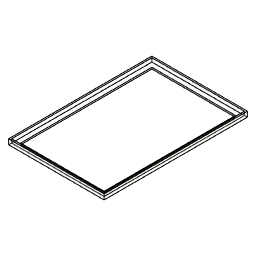
SafetyMachineCase (Autodesk Fusion 360 archive; units mm, degrees)
design "cover"
Autodesk Fusion 360 part; units mm, degrees
(part 1 of 2)
sketch "スケッチ1" plane through (0, 0, 0) normal (0, 0, 1) x (1, 0, 0)
  line L0 (31, 47) -> (-31, 47)
  line L1 (-31, 47) -> (-31, -47)
  line L2 (-31, -47) -> (31, -47)
  line L3 (31, -47) -> (31, 47)
  line L4 (31, 47) -> (-31, -47) construction
  line L5 (-31, 47) -> (31, -47) construction
  line L6 (-32, 48) -> (-32, -48)
  line L7 (-32, -48) -> (32, -48)
  line L8 (32, -48) -> (32, 48)
  line L9 (32, 48) -> (-32, 48)
  line L10 (-28, 44) -> (-28, -44)
  line L11 (-28, -44) -> (28, -44)
  line L12 (28, -44) -> (28, 44)
  line L13 (28, 44) -> (-28, 44)
  dimension "d1" = 62
  dimension "d2" = 94
  dimension "d3" = 1
  dimension "d4" = -3
  constraint horizontal L0
  constraint perpendicular L0 L1
  constraint parallel L0 L2
  constraint parallel L1 L3
  constraint coincident L4 origin
  constraint coincident L5 origin
  measures "d1" distance of L0.start L0.end
  measures "d2" distance of L0.start L2.end
extrude "押し出し1" add sketch "スケッチ1" along normal blind 2.5 contours L6 L7 L8 L9
extrude "押し出し2" add sketch "スケッチ1" against normal blind 1 contours L0 L1 L2 L3 | L6 L7 L8 L9

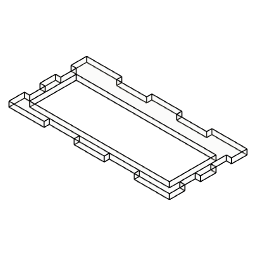
design "migisokumen"
Autodesk Fusion 360 part; units mm, degrees
sketch "スケッチ1" plane through (0, 0, 0) normal (0, 0, 1) x (1, 0, 0)
  line L0 (31, 15) -> (-31, 15)
  line L1 (-31, 15) -> (-31, -15)
  line L2 (-31, -15) -> (31, -15)
  line L3 (31, -15) -> (31, 15)
  line L4 (31, 15) -> (-31, -15) construction
  line L5 (-31, 15) -> (31, -15) construction
  dimension "d1" = 62
  dimension "d2" = 30
  constraint horizontal L0
  constraint perpendicular L0 L1
  constraint parallel L0 L2
  constraint parallel L1 L3
  constraint coincident L4 origin
  constraint coincident L5 origin
  measures "d1" distance of L0.start L0.end
  measures "d2" distance of L0.end L1.end
extrude "押し出し1" add sketch "スケッチ1" along normal blind 2
sketch "スケッチ2" plane through (0, 0, 0) normal (0, 0, 1) x (1, 0, 0)
  line L0 (31, 9) -> (29, 9)
  line L1 (29, 9) -> (29, 3)
  line L2 (29, 3) -> (31, 3)
  line L3 (31, 3) -> (31, 9)
  line L4 (31, -15) -> (31, 15)
  line L5 (0, 0) -> (48, 0)
  line L6 (31, -3) -> (31, -9)
  line L7 (29, -3) -> (31, -3)
  line L8 (29, -9) -> (29, -3)
  line L9 (31, -9) -> (29, -9)
  line L10 (0, 0) -> (0, -25)
  line L11 (-31, 9) -> (-29, 9)
  line L12 (-31, 3) -> (-31, 9)
  line L13 (-29, -3) -> (-31, -3)
  line L14 (-31, -3) -> (-31, -9)
  line L15 (-31, -9) -> (-29, -9)
  line L16 (-29, -9) -> (-29, -3)
  line L17 (-29, 3) -> (-31, 3)
  line L18 (-29, 9) -> (-29, 3)
  dimension "d9" = 6
  dimension "d10" = 3
  dimension "d23" = 2
  constraint horizontal L0
  constraint vertical L1
  constraint horizontal L2
  constraint vertical L3
  constraint collinear L3 L4
  constraint coincident L5.start L10.start
  constraint perpendicular L4 L5
  constraint symmetric L0.start L5 L6.end
  constraint symmetric L0.end L5 L8.start
  constraint symmetric L1.end L5 L7.start
  constraint symmetric L2.end L5 L6.start
  constraint perpendicular L5 L10
  constraint symmetric L0.start L10 L11.start
  constraint symmetric L0.end L10 L11.end
  constraint symmetric L1.end L10 L17.start
  constraint symmetric L2.end L10 L12.start
  constraint symmetric L8.start L10 L15.end
  constraint symmetric L6.end L10 L14.end
  constraint symmetric L6.start L10 L13.end
  constraint symmetric L7.start L10 L13.start
  measures "d9" distance of L0.end L1.end
  measures "d10" distance of L5.start L2
  measures "d23" distance of L1 L3
extrude "押し出し2" cut sketch "スケッチ2" along normal up to surface (2 mm away)
sketch "スケッチ3" plane through (0, 0, 2) normal (0, 0, 1) x (-1, 0, 0)
  line L0 (-31, 3) -> (-31, -3)
  line L1 (-31, -15) -> (31, -15)
  line L2 (31, -15) -> (31, -9)
  line L3 (17.4, -15) -> (5.8, -15)
  line L4 (5.8, -15) -> (5.8, -13)
  line L5 (5.8, -13) -> (17.4, -13)
  line L6 (17.4, -13) -> (17.4, -15)
  line L7 (0, 0) -> (0, -10)
  line L8 (0, 0) -> (9, 0)
  line L9 (-17.4, -15) -> (-5.8, -15)
  line L10 (-5.8, -15) -> (-5.8, -13)
  line L11 (-17.4, -13) -> (-17.4, -15)
  line L12 (-5.8, -13) -> (-17.4, -13)
  line L13 (-5.8, 15) -> (-5.8, 13)
  line L14 (-17.4, 13) -> (-17.4, 15)
  line L15 (17.4, 15) -> (5.8, 15)
  line L16 (5.8, 13) -> (17.4, 13)
  line L17 (-17.4, 15) -> (-5.8, 15)
  line L18 (-5.8, 13) -> (-17.4, 13)
  line L19 (5.8, 15) -> (5.8, 13)
  line L20 (17.4, 13) -> (17.4, 15)
  line L21 (-31, 9) -> (-29, 9)
  line L22 (-29, 9) -> (-29, 3)
  line L23 (-29, 3) -> (-31, 3)
  line L24 (-31, -3) -> (-29, -3)
  line L25 (-29, -3) -> (-29, -9)
  line L26 (-29, -9) -> (-31, -9)
  line L27 (-31, -9) -> (-31, -15)
  line L28 (31, -9) -> (29, -9)
  line L29 (29, -9) -> (29, -3)
  line L30 (29, -3) -> (31, -3)
  line L31 (31, -3) -> (31, 3)
  line L32 (31, 3) -> (29, 3)
  line L33 (29, 3) -> (29, 9)
  line L34 (29, 9) -> (31, 9)
  line L35 (31, 9) -> (31, 15)
  line L36 (-31, 15) -> (-31, 9)
  dimension "d16" = 11.6
  dimension "d21" = 2
  dimension "d22" = 5.8
  constraint horizontal L3
  constraint vertical L4
  constraint horizontal L5
  constraint vertical L6
  constraint coincident L1 L3.start
  constraint coincident L7.start L8.start
  constraint parallel L4 L7
  constraint perpendicular L7 L8
  constraint symmetric L3.start L7 L9.start
  constraint symmetric L3.end L7 L9.end
  constraint symmetric L4.end L7 L10.end
  constraint symmetric L5.end L7 L11.start
  constraint symmetric L3.start L8 L15.start
  constraint symmetric L3.end L8 L15.end
  constraint symmetric L4.end L8 L16.start
  constraint symmetric L5.end L8 L16.end
  constraint symmetric L8 L9.start L14.end
  constraint symmetric L8 L9.end L13.start
  constraint symmetric L8 L11.start L14.start
  constraint symmetric L8 L10.end L13.end
  measures "d16" distance of L4.end L5.end
  measures "d21" distance of L1 L5
  measures "d22" distance of L7.start L4
extrude "押し出し3" cut sketch "スケッチ3" against normal up to surface (2 mm away)
sketch "スケッチ4" plane through (0, 0, 2) normal (0, 0, 1) x (-1, 0, 0)
  line L0 (-17.4, -15) -> (-17.4, -13)
  line L1 (-17.4, -13) -> (-5.8, -13)
  line L2 (-5.8, -13) -> (-5.8, -15)
  line L3 (-5.8, -15) -> (5.8, -15)
  line L4 (5.8, -15) -> (5.8, -13)
  line L5 (5.8, -13) -> (17.4, -13)
  line L6 (17.4, -13) -> (17.4, -15)
  line L7 (17.4, -15) -> (31, -15)
  line L8 (31, -15) -> (31, -9)
  line L9 (31, -9) -> (29, -9)
  line L10 (29, -9) -> (29, -3)
  line L11 (29, -3) -> (31, -3)
  line L12 (31, -3) -> (31, 3)
  line L13 (31, 3) -> (29, 3)
  line L14 (29, 3) -> (29, 9)
  line L15 (29, 9) -> (31, 9)
  line L16 (31, 9) -> (31, 15)
  line L17 (31, 15) -> (17.4, 15)
  line L18 (17.4, 15) -> (17.4, 13)
  line L19 (17.4, 13) -> (5.8, 13)
  line L20 (5.8, 13) -> (5.8, 15)
  line L21 (5.8, 15) -> (-5.8, 15)
  line L22 (-5.8, 15) -> (-5.8, 13)
  line L23 (-5.8, 13) -> (-17.4, 13)
  line L24 (-17.4, 13) -> (-17.4, 15)
  line L25 (-17.4, 15) -> (-31, 15)
  line L26 (-31, 15) -> (-31, 9)
  line L27 (-31, 9) -> (-29, 9)
  line L28 (-29, 9) -> (-29, 3)
  line L29 (-29, 3) -> (-31, 3)
  line L30 (-31, 3) -> (-31, -3)
  line L31 (-31, -3) -> (-29, -3)
  line L32 (-29, -3) -> (-29, -9)
  line L33 (-29, -9) -> (-31, -9)
  line L34 (-31, -9) -> (-31, -15)
  line L35 (-31, -15) -> (-17.4, -15)
  line L36 (27, 11) -> (-27, 11)
  line L37 (-27, 11) -> (-27, -7)
  line L38 (-27, -7) -> (27, -7)
  line L39 (27, -7) -> (27, 11)
  dimension "d24" = 54
  dimension "d25" = 27
  dimension "d26" = 2
  dimension "d27" = 18
  constraint horizontal L36
  constraint vertical L37
  constraint horizontal L38
  constraint vertical L39
  measures "d24" distance of L37.end L38.end
  measures "d25" distance of origin L37
  measures "d26" distance of L19 L36
  measures "d27" distance of L36.start L38.end
extrude "押し出し4" cut sketch "スケッチ4" against normal up to surface (2 mm away) contours L36 L37 L38 L39
equation "d1 = 58 mm + t * 2"
equation "d3 = t"
equation "t = 2 mm" comment "板厚"
equation "w = 11.6 mm" comment "かみ合い幅"
equation "d9 = w3"
equation "d10 = w3 / 2"
equation "w2 = 18 mm"
equation "w3 = 6 mm"
equation "d16 = w"
equation "d21 = t"
equation "d22 = w / 2"
equation "d23 = t"
equation "d25 = ( 54 / 2 ) * 1 mm"

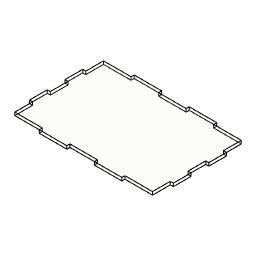
design "joumen"
Autodesk Fusion 360 part; units mm, degrees
sketch "スケッチ1" plane through (0, 0, 0) normal (0, 0, 1) x (1, 0, 0)
  line L0 (45, 29) -> (-45, 29)
  line L1 (-45, 29) -> (-45, -29)
  line L2 (-45, -29) -> (45, -29)
  line L3 (45, -29) -> (45, 29)
  line L4 (45, 29) -> (-45, -29) construction
  line L5 (-45, 29) -> (45, -29) construction
  dimension "d1" = 90
  dimension "d2" = 58
  constraint horizontal L0
  constraint perpendicular L0 L1
  constraint parallel L0 L2
  constraint parallel L1 L3
  constraint coincident L4 origin
  constraint coincident L5 origin
  measures "d1" distance of L0.start L0.end
  measures "d2" distance of L0.end L1.end
extrude "押し出し1" add sketch "スケッチ1" along normal blind 2
sketch "スケッチ2" plane through (0, 0, 0) normal (0, 0, 1) x (1, 0, 0)
  line L0 (45, 17.4) -> (47, 17.4)
  line L1 (47, 17.4) -> (47, 5.8)
  line L2 (47, 5.8) -> (45, 5.8)
  line L3 (45, 5.8) -> (45, 17.4)
  line L4 (45, -29) -> (45, 29)
  line L5 (0, 0) -> (48, 0)
  line L6 (45, -5.8) -> (45, -17.4)
  line L7 (47, -5.8) -> (45, -5.8)
  line L8 (47, -17.4) -> (47, -5.8)
  line L9 (45, -17.4) -> (47, -17.4)
  line L10 (0, 0) -> (0, -25)
  line L11 (-45, 17.4) -> (-47, 17.4)
  line L12 (-45, 5.8) -> (-45, 17.4)
  line L13 (-47, -5.8) -> (-45, -5.8)
  line L14 (-45, -5.8) -> (-45, -17.4)
  line L15 (-45, -17.4) -> (-47, -17.4)
  line L16 (-47, -17.4) -> (-47, -5.8)
  line L17 (-47, 5.8) -> (-45, 5.8)
  line L18 (-47, 17.4) -> (-47, 5.8)
  dimension "d6" = 2
  dimension "d9" = 11.6
  dimension "d10" = 5.8
  constraint horizontal L0
  constraint vertical L1
  constraint horizontal L2
  constraint vertical L3
  constraint collinear L3 L4
  constraint coincident L5.start L10.start
  constraint perpendicular L4 L5
  constraint symmetric L0.start L5 L6.end
  constraint symmetric L0.end L5 L8.start
  constraint symmetric L1.end L5 L7.start
  constraint symmetric L2.end L5 L6.start
  constraint perpendicular L5 L10
  constraint symmetric L0.start L10 L11.start
  constraint symmetric L0.end L10 L11.end
  constraint symmetric L1.end L10 L17.start
  constraint symmetric L2.end L10 L12.start
  constraint symmetric L8.start L10 L15.end
  constraint symmetric L6.end L10 L14.end
  constraint symmetric L6.start L10 L13.end
  constraint symmetric L7.start L10 L13.start
  measures "d6" distance of L0.start L0.end
  measures "d9" distance of L0.end L1.end
  measures "d10" distance of L5.start L2
extrude "押し出し2" add sketch "スケッチ2" along normal up to surface (2 mm away)
sketch "スケッチ3" plane through (0, 0, 2) normal (0, 0, 1) x (-1, 0, 0)
  line L0 (-45, 29) -> (-45, 17.4)
  line L1 (-45, 17.4) -> (-47, 17.4)
  line L2 (-47, 17.4) -> (-47, 5.8)
  line L3 (-47, 5.8) -> (-45, 5.8)
  line L4 (-45, 5.8) -> (-45, -5.8)
  line L5 (-45, -5.8) -> (-47, -5.8)
  line L6 (-47, -5.8) -> (-47, -17.4)
  line L7 (-47, -17.4) -> (-45, -17.4)
  line L8 (-45, -17.4) -> (-45, -29)
  line L9 (-45, -29) -> (45, -29)
  line L10 (45, -29) -> (45, -17.4)
  line L11 (45, -17.4) -> (47, -17.4)
  line L12 (47, -17.4) -> (47, -5.8)
  line L13 (47, -5.8) -> (45, -5.8)
  line L14 (45, -5.8) -> (45, 5.8)
  line L15 (45, 5.8) -> (47, 5.8)
  line L16 (47, 5.8) -> (47, 17.4)
  line L17 (47, 17.4) -> (45, 17.4)
  line L18 (45, 17.4) -> (45, 29)
  line L19 (45, 29) -> (-45, 29)
  line L20 (27, -29) -> (9, -29)
  line L21 (9, -29) -> (9, -31)
  line L22 (9, -31) -> (27, -31)
  line L23 (27, -31) -> (27, -29)
  line L24 (0, 0) -> (0, -29)
  line L25 (-27, -31) -> (-27, -29)
  line L26 (-9, -31) -> (-27, -31)
  line L27 (-9, -29) -> (-9, -31)
  line L28 (-27, -29) -> (-9, -29)
  line L29 (0, 0) -> (45, 0)
  line L30 (9, 31) -> (27, 31)
  line L31 (-27, 29) -> (-9, 29)
  line L32 (9, 29) -> (9, 31)
  line L33 (-27, 31) -> (-27, 29)
  line L34 (27, 29) -> (9, 29)
  line L35 (-9, 29) -> (-9, 31)
  line L36 (-9, 31) -> (-27, 31)
  line L37 (27, 31) -> (27, 29)
  point P0 (0, 29)
  dimension "d16" = 18
  dimension "d17" = 9
  dimension "d18" = 2
  constraint horizontal L20
  constraint vertical L21
  constraint horizontal L22
  constraint vertical L23
  constraint coincident L9 L20.start
  constraint coincident L24.start L29.start
  constraint midpoint L9 L24.end
  constraint symmetric L20.start L24 L25.end
  constraint symmetric L20.end L24 L27.start
  constraint symmetric L21.end L24 L26.start
  constraint symmetric L22.end L24 L25.start
  constraint midpoint L14 L29.end
  constraint symmetric L20.start L29 L34.start
  constraint symmetric L20.end L29 L32.start
  constraint symmetric L21.end L29 L30.start
  constraint symmetric L22.end L29 L30.end
  constraint symmetric L24.end L29 P0
  constraint symmetric L26.start L29 L35.end
  constraint symmetric L27.start L29 L31.end
  constraint symmetric L25.start L29 L33.start
  constraint symmetric L25.end L29 L31.start
  measures "d16" distance of L21.end L22.end
  measures "d17" distance of L24.start L21
  measures "d18" distance of L20.start L22.end
extrude "押し出し3" add sketch "スケッチ3" against normal up to surface (2 mm away) contours L19 L31 L33 L35 L36 | L19 L30 L32 L34 L37 | L9 L25 L26 L27 L28 | L9 L20 L21 L22 L23
equation "d3 = t"
equation "t = 2 mm" comment "板厚"
equation "d6 = t"
equation "w = 11.6 mm" comment "かみ合い幅"
equation "d9 = w"
equation "d10 = w / 2"
equation "w2 = 18 mm"
equation "w3 = 6 mm"
equation "d16 = w2"
equation "d17 = w2 / 2"
equation "d18 = t"

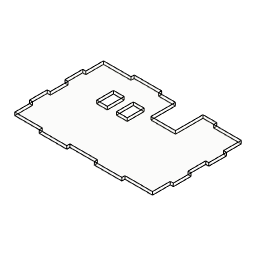
design "joumen_ishole"
Autodesk Fusion 360 part; units mm, degrees
sketch "スケッチ1" plane through (0, 0, 0) normal (0, 0, 1) x (1, 0, 0)
  line L0 (45, 29) -> (-45, 29)
  line L1 (-45, 29) -> (-45, -29)
  line L2 (-45, -29) -> (45, -29)
  line L3 (45, -29) -> (45, 29)
  line L4 (45, 29) -> (-45, -29) construction
  line L5 (-45, 29) -> (45, -29) construction
  dimension "d1" = 90
  dimension "d2" = 58
  constraint horizontal L0
  constraint perpendicular L0 L1
  constraint parallel L0 L2
  constraint parallel L1 L3
  constraint coincident L4 origin
  constraint coincident L5 origin
  measures "d1" distance of L0.start L0.end
  measures "d2" distance of L0.end L1.end
extrude "押し出し1" add sketch "スケッチ1" along normal blind 2
sketch "スケッチ2" plane through (0, 0, 0) normal (0, 0, 1) x (1, 0, 0)
  line L0 (45, 17.4) -> (47, 17.4)
  line L1 (47, 17.4) -> (47, 5.8)
  line L2 (47, 5.8) -> (45, 5.8)
  line L3 (45, 5.8) -> (45, 17.4)
  line L4 (45, -29) -> (45, 29)
  line L5 (0, 0) -> (48, 0)
  line L6 (45, -5.8) -> (45, -17.4)
  line L7 (47, -5.8) -> (45, -5.8)
  line L8 (47, -17.4) -> (47, -5.8)
  line L9 (45, -17.4) -> (47, -17.4)
  line L10 (0, 0) -> (0, -25)
  line L11 (-45, 17.4) -> (-47, 17.4)
  line L12 (-45, 5.8) -> (-45, 17.4)
  line L13 (-47, -5.8) -> (-45, -5.8)
  line L14 (-45, -5.8) -> (-45, -17.4)
  line L15 (-45, -17.4) -> (-47, -17.4)
  line L16 (-47, -17.4) -> (-47, -5.8)
  line L17 (-47, 5.8) -> (-45, 5.8)
  line L18 (-47, 17.4) -> (-47, 5.8)
  dimension "d6" = 2
  dimension "d9" = 11.6
  dimension "d10" = 5.8
  constraint horizontal L0
  constraint vertical L1
  constraint horizontal L2
  constraint vertical L3
  constraint collinear L3 L4
  constraint coincident L5.start L10.start
  constraint perpendicular L4 L5
  constraint symmetric L0.start L5 L6.end
  constraint symmetric L0.end L5 L8.start
  constraint symmetric L1.end L5 L7.start
  constraint symmetric L2.end L5 L6.start
  constraint perpendicular L5 L10
  constraint symmetric L0.start L10 L11.start
  constraint symmetric L0.end L10 L11.end
  constraint symmetric L1.end L10 L17.start
  constraint symmetric L2.end L10 L12.start
  constraint symmetric L8.start L10 L15.end
  constraint symmetric L6.end L10 L14.end
  constraint symmetric L6.start L10 L13.end
  constraint symmetric L7.start L10 L13.start
  measures "d6" distance of L0.start L0.end
  measures "d9" distance of L0.end L1.end
  measures "d10" distance of L5.start L2
extrude "押し出し2" add sketch "スケッチ2" along normal up to surface (2 mm away)
sketch "スケッチ3" plane through (0, 0, 2) normal (0, 0, 1) x (-1, 0, 0)
  line L0 (-45, 29) -> (-45, 17.4)
  line L1 (-45, 17.4) -> (-47, 17.4)
  line L2 (-47, 17.4) -> (-47, 5.8)
  line L3 (-47, 5.8) -> (-45, 5.8)
  line L4 (-45, 5.8) -> (-45, -5.8)
  line L5 (-45, -5.8) -> (-47, -5.8)
  line L6 (-47, -5.8) -> (-47, -17.4)
  line L7 (-47, -17.4) -> (-45, -17.4)
  line L8 (-45, -17.4) -> (-45, -29)
  line L9 (-45, -29) -> (45, -29)
  line L10 (45, -29) -> (45, -17.4)
  line L11 (45, -17.4) -> (47, -17.4)
  line L12 (47, -17.4) -> (47, -5.8)
  line L13 (47, -5.8) -> (45, -5.8)
  line L14 (45, -5.8) -> (45, 5.8)
  line L15 (45, 5.8) -> (47, 5.8)
  line L16 (47, 5.8) -> (47, 17.4)
  line L17 (47, 17.4) -> (45, 17.4)
  line L18 (45, 17.4) -> (45, 29)
  line L19 (45, 29) -> (-45, 29)
  line L20 (27, -29) -> (9, -29)
  line L21 (9, -29) -> (9, -31)
  line L22 (9, -31) -> (27, -31)
  line L23 (27, -31) -> (27, -29)
  line L24 (0, 0) -> (0, -29)
  line L25 (-27, -31) -> (-27, -29)
  line L26 (-9, -31) -> (-27, -31)
  line L27 (-9, -29) -> (-9, -31)
  line L28 (-27, -29) -> (-9, -29)
  line L29 (0, 0) -> (45, 0)
  line L30 (9, 31) -> (27, 31)
  line L31 (-27, 29) -> (-9, 29)
  line L32 (9, 29) -> (9, 31)
  line L33 (-27, 31) -> (-27, 29)
  line L34 (27, 29) -> (9, 29)
  line L35 (-9, 29) -> (-9, 31)
  line L36 (-9, 31) -> (-27, 31)
  line L37 (27, 31) -> (27, 29)
  point P0 (0, 29)
  dimension "d16" = 18
  dimension "d17" = 9
  dimension "d18" = 2
  constraint horizontal L20
  constraint vertical L21
  constraint horizontal L22
  constraint vertical L23
  constraint coincident L9 L20.start
  constraint coincident L24.start L29.start
  constraint midpoint L9 L24.end
  constraint symmetric L20.start L24 L25.end
  constraint symmetric L20.end L24 L27.start
  constraint symmetric L21.end L24 L26.start
  constraint symmetric L22.end L24 L25.start
  constraint midpoint L14 L29.end
  constraint symmetric L20.start L29 L34.start
  constraint symmetric L20.end L29 L32.start
  constraint symmetric L21.end L29 L30.start
  constraint symmetric L22.end L29 L30.end
  constraint symmetric L24.end L29 P0
  constraint symmetric L26.start L29 L35.end
  constraint symmetric L27.start L29 L31.end
  constraint symmetric L25.start L29 L33.start
  constraint symmetric L25.end L29 L31.start
  measures "d16" distance of L21.end L22.end
  measures "d17" distance of L24.start L21
  measures "d18" distance of L20.start L22.end
extrude "押し出し3" add sketch "スケッチ3" against normal up to surface (2 mm away) contours L19 L31 L33 L35 L36 | L19 L30 L32 L34 L37 | L9 L25 L26 L27 L28 | L9 L20 L21 L22 L23
sketch "スケッチ4" plane through (0, 0, 2) normal (0, 0, 1) x (-1, 0, 0)
  line L0 (-45, 29) -> (-45, 17.4)
  line L1 (-45, 17.4) -> (-47, 17.4)
  line L2 (-47, 17.4) -> (-47, 5.8)
  line L3 (-47, 5.8) -> (-45, 5.8)
  line L4 (-45, 5.8) -> (-45, -5.8)
  line L5 (-45, -5.8) -> (-47, -5.8)
  line L6 (-47, -5.8) -> (-47, -17.4)
  line L7 (-47, -17.4) -> (-45, -17.4)
  line L8 (-45, -17.4) -> (-45, -29)
  line L9 (-45, -29) -> (-27, -29)
  line L10 (-27, -29) -> (-27, -31)
  line L11 (-27, -31) -> (-9, -31)
  line L12 (-9, -31) -> (-9, -29)
  line L13 (-9, -29) -> (9, -29)
  line L14 (9, -29) -> (9, -31)
  line L15 (9, -31) -> (27, -31)
  line L16 (27, -31) -> (27, -29)
  line L17 (27, -29) -> (45, -29)
  line L18 (45, -29) -> (45, -17.4)
  line L19 (45, -17.4) -> (47, -17.4)
  line L20 (47, -17.4) -> (47, -5.8)
  line L21 (47, -5.8) -> (45, -5.8)
  line L22 (45, -5.8) -> (45, 5.8)
  line L23 (45, 5.8) -> (47, 5.8)
  line L24 (47, 5.8) -> (47, 17.4)
  line L25 (47, 17.4) -> (45, 17.4)
  line L26 (45, 17.4) -> (45, 29)
  line L27 (45, 29) -> (27, 29)
  line L28 (27, 29) -> (27, 31)
  line L29 (27, 31) -> (9, 31)
  line L30 (9, 31) -> (9, 29)
  line L31 (9, 29) -> (-9, 29)
  line L32 (-9, 29) -> (-9, 31)
  line L33 (-9, 31) -> (-27, 31)
  line L34 (-27, 31) -> (-27, 29)
  line L35 (-27, 29) -> (-45, 29)
  line L36 (25, -15.5) -> (18, -15.5)
  line L37 (18, -15.5) -> (18, -4.5)
  line L38 (18, -4.5) -> (25, -4.5)
  line L39 (25, -4.5) -> (25, -15.5)
  line L40 (12, -15.5) -> (5, -15.5)
  line L41 (5, -15.5) -> (5, -4.5)
  line L42 (5, -4.5) -> (12, -4.5)
  line L43 (12, -4.5) -> (12, -15.5)
  dimension "d21" = 7
  dimension "d22" = 11
  dimension "d23" = 50
  dimension "d24" = 6
  dimension "d25" = 13.5
  constraint horizontal L36
  constraint vertical L37
  constraint horizontal L38
  constraint vertical L39
  constraint horizontal L40
  constraint vertical L41
  constraint horizontal L42
  constraint vertical L43
  constraint equal L36 L40
  constraint equal L39 L43
  constraint collinear L36 L40
  measures "d21" distance of L36.start L36.end
  measures "d22" distance of L36.start L38.end
  measures "d23" distance of L8 L41
  measures "d24" distance of L37 L43
  measures "d25" distance of L9 L40
extrude "押し出し4" cut sketch "スケッチ4" against normal up to surface (2 mm away) contours L36 L37 L38 L39 | L40 L41 L42 L43
sketch "スケッチ5" plane through (0, 0, 2) normal (0, 0, 1) x (-1, 0, 0)
  line L0 (25, -4.5) -> (25, -15.5)
  line L1 (25, -15.5) -> (18, -15.5)
  line L2 (18, -15.5) -> (18, -4.5)
  line L3 (18, -4.5) -> (25, -4.5)
  line L4 (12, -4.5) -> (12, -15.5)
  line L5 (12, -15.5) -> (5, -15.5)
  line L6 (5, -15.5) -> (5, -4.5)
  line L7 (5, -4.5) -> (12, -4.5)
  line L8 (-45, 29) -> (-45, 17.4)
  line L9 (-45, 17.4) -> (-47, 17.4)
  line L10 (-47, 17.4) -> (-47, 5.8)
  line L11 (-47, 5.8) -> (-45, 5.8)
  line L12 (-45, 5.8) -> (-45, -5.8)
  line L13 (-45, -5.8) -> (-47, -5.8)
  line L14 (-47, -5.8) -> (-47, -17.4)
  line L15 (-47, -17.4) -> (-45, -17.4)
  line L16 (-45, -17.4) -> (-45, -29)
  line L17 (-45, -29) -> (-27, -29)
  line L18 (-27, -29) -> (-27, -31)
  line L19 (-27, -31) -> (-9, -31)
  line L20 (-9, -31) -> (-9, -29)
  line L21 (-9, -29) -> (9, -29)
  line L22 (9, -29) -> (9, -31)
  line L23 (9, -31) -> (27, -31)
  line L24 (27, -31) -> (27, -29)
  line L25 (27, -29) -> (45, -29)
  line L26 (45, -29) -> (45, -17.4)
  line L27 (45, -17.4) -> (47, -17.4)
  line L28 (47, -17.4) -> (47, -5.8)
  line L29 (47, -5.8) -> (45, -5.8)
  line L30 (45, -5.8) -> (45, 5.8)
  line L31 (45, 5.8) -> (47, 5.8)
  line L32 (47, 5.8) -> (47, 17.4)
  line L33 (47, 17.4) -> (45, 17.4)
  line L34 (45, 17.4) -> (45, 29)
  line L35 (45, 29) -> (27, 29)
  line L36 (27, 29) -> (27, 31)
  line L37 (27, 31) -> (9, 31)
  line L38 (9, 31) -> (9, 29)
  line L39 (9, 29) -> (-9, 29)
  line L40 (-9, 29) -> (-9, 31)
  line L41 (-9, 31) -> (-27, 31)
  line L42 (-27, 31) -> (-27, 29)
  line L43 (-27, 29) -> (-45, 29)
  line L44 (-2, -13) -> (-18, -13)
  line L45 (-18, -13) -> (-18, -31)
  line L46 (-18, -31) -> (-2, -31)
  line L47 (-2, -31) -> (-2, -13)
  dimension "d29" = 16
  dimension "d30" = 7
  dimension "d33" = 18
  constraint vertical L45
  constraint horizontal L46
  constraint vertical L47
  constraint collinear L19 L46
  measures "d29" distance of L45.end L46.end
  measures "d30" distance of L6 L47
  measures "d33" distance of L44 L46
extrude "押し出し5" cut sketch "スケッチ5" against normal up to surface (2 mm away) contours L19 L20 L21 L44 L45 L46 L47
equation "d3 = t"
equation "t = 2 mm" comment "板厚"
equation "d6 = t"
equation "w = 11.6 mm" comment "かみ合い幅"
equation "d9 = w"
equation "d10 = w / 2"
equation "w2 = 18 mm"
equation "w3 = 6 mm"
equation "d16 = w2"
equation "d17 = w2 / 2"
equation "d18 = t"

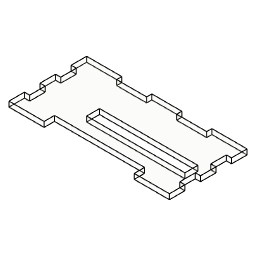
design "hidarisokumen"
Autodesk Fusion 360 part; units mm, degrees
sketch "スケッチ1" plane through (0, 0, 0) normal (0, 0, 1) x (1, 0, 0)
  line L0 (31, 15) -> (-31, 15)
  line L1 (-31, 15) -> (-31, -15)
  line L2 (-31, -15) -> (31, -15)
  line L3 (31, -15) -> (31, 15)
  line L4 (31, 15) -> (-31, -15) construction
  line L5 (-31, 15) -> (31, -15) construction
  dimension "d1" = 62
  dimension "d2" = 30
  constraint horizontal L0
  constraint perpendicular L0 L1
  constraint parallel L0 L2
  constraint parallel L1 L3
  constraint coincident L4 origin
  constraint coincident L5 origin
  measures "d1" distance of L0.start L0.end
  measures "d2" distance of L0.end L1.end
extrude "押し出し1" add sketch "スケッチ1" along normal blind 2
sketch "スケッチ2" plane through (0, 0, 0) normal (0, 0, 1) x (1, 0, 0)
  line L0 (31, 9) -> (29, 9)
  line L1 (29, 9) -> (29, 3)
  line L2 (29, 3) -> (31, 3)
  line L3 (31, 3) -> (31, 9)
  line L4 (31, -15) -> (31, 15)
  line L5 (0, 0) -> (48, 0)
  line L6 (31, -3) -> (31, -9)
  line L7 (29, -3) -> (31, -3)
  line L8 (29, -9) -> (29, -3)
  line L9 (31, -9) -> (29, -9)
  line L10 (0, 0) -> (0, -25)
  line L11 (-31, 9) -> (-29, 9)
  line L12 (-31, 3) -> (-31, 9)
  line L13 (-29, -3) -> (-31, -3)
  line L14 (-31, -3) -> (-31, -9)
  line L15 (-31, -9) -> (-29, -9)
  line L16 (-29, -9) -> (-29, -3)
  line L17 (-29, 3) -> (-31, 3)
  line L18 (-29, 9) -> (-29, 3)
  dimension "d9" = 6
  dimension "d10" = 3
  dimension "d23" = 2
  constraint horizontal L0
  constraint vertical L1
  constraint horizontal L2
  constraint vertical L3
  constraint collinear L3 L4
  constraint coincident L5.start L10.start
  constraint perpendicular L4 L5
  constraint symmetric L0.start L5 L6.end
  constraint symmetric L0.end L5 L8.start
  constraint symmetric L1.end L5 L7.start
  constraint symmetric L2.end L5 L6.start
  constraint perpendicular L5 L10
  constraint symmetric L0.start L10 L11.start
  constraint symmetric L0.end L10 L11.end
  constraint symmetric L1.end L10 L17.start
  constraint symmetric L2.end L10 L12.start
  constraint symmetric L8.start L10 L15.end
  constraint symmetric L6.end L10 L14.end
  constraint symmetric L6.start L10 L13.end
  constraint symmetric L7.start L10 L13.start
  measures "d9" distance of L0.end L1.end
  measures "d10" distance of L5.start L2
  measures "d23" distance of L1 L3
extrude "押し出し2" cut sketch "スケッチ2" along normal up to surface (2 mm away)
sketch "スケッチ3" plane through (0, 0, 2) normal (0, 0, 1) x (-1, 0, 0)
  line L0 (-31, 3) -> (-31, -3)
  line L1 (-31, -15) -> (31, -15)
  line L2 (31, -15) -> (31, -9)
  line L3 (17.4, -15) -> (5.8, -15)
  line L4 (5.8, -15) -> (5.8, -13)
  line L5 (5.8, -13) -> (17.4, -13)
  line L6 (17.4, -13) -> (17.4, -15)
  line L7 (0, 0) -> (0, -10)
  line L8 (0, 0) -> (9, 0)
  line L9 (-17.4, -15) -> (-5.8, -15)
  line L10 (-5.8, -15) -> (-5.8, -13)
  line L11 (-17.4, -13) -> (-17.4, -15)
  line L12 (-5.8, -13) -> (-17.4, -13)
  line L13 (-5.8, 15) -> (-5.8, 13)
  line L14 (-17.4, 13) -> (-17.4, 15)
  line L15 (17.4, 15) -> (5.8, 15)
  line L16 (5.8, 13) -> (17.4, 13)
  line L17 (-17.4, 15) -> (-5.8, 15)
  line L18 (-5.8, 13) -> (-17.4, 13)
  line L19 (5.8, 15) -> (5.8, 13)
  line L20 (17.4, 13) -> (17.4, 15)
  line L21 (-31, 9) -> (-29, 9)
  line L22 (-29, 9) -> (-29, 3)
  line L23 (-29, 3) -> (-31, 3)
  line L24 (-31, -3) -> (-29, -3)
  line L25 (-29, -3) -> (-29, -9)
  line L26 (-29, -9) -> (-31, -9)
  line L27 (-31, -9) -> (-31, -15)
  line L28 (31, -9) -> (29, -9)
  line L29 (29, -9) -> (29, -3)
  line L30 (29, -3) -> (31, -3)
  line L31 (31, -3) -> (31, 3)
  line L32 (31, 3) -> (29, 3)
  line L33 (29, 3) -> (29, 9)
  line L34 (29, 9) -> (31, 9)
  line L35 (31, 9) -> (31, 15)
  line L36 (-31, 15) -> (-31, 9)
  dimension "d16" = 11.6
  dimension "d21" = 2
  dimension "d22" = 5.8
  constraint horizontal L3
  constraint vertical L4
  constraint horizontal L5
  constraint vertical L6
  constraint coincident L1 L3.start
  constraint coincident L7.start L8.start
  constraint parallel L4 L7
  constraint perpendicular L7 L8
  constraint symmetric L3.start L7 L9.start
  constraint symmetric L3.end L7 L9.end
  constraint symmetric L4.end L7 L10.end
  constraint symmetric L5.end L7 L11.start
  constraint symmetric L3.start L8 L15.start
  constraint symmetric L3.end L8 L15.end
  constraint symmetric L4.end L8 L16.start
  constraint symmetric L5.end L8 L16.end
  constraint symmetric L8 L9.start L14.end
  constraint symmetric L8 L9.end L13.start
  constraint symmetric L8 L11.start L14.start
  constraint symmetric L8 L10.end L13.end
  measures "d16" distance of L4.end L5.end
  measures "d21" distance of L1 L5
  measures "d22" distance of L7.start L4
extrude "押し出し3" cut sketch "スケッチ3" against normal up to surface (2 mm away)
sketch "スケッチ4" plane through (0, -15, 0) normal (0, -1, 0) x (1, 0, 0)
  line L0 (-5.8, 2) -> (-5.8, 0)
  line L1 (-5.8, 0) -> (5.8, 0)
  line L2 (5.8, 0) -> (5.8, 2)
  line L3 (5.8, 2) -> (-5.8, 2)
extrude "押し出し4" cut sketch "スケッチ4" against normal blind 2
sketch "スケッチ5" plane through (0, 0, 2) normal (0, 0, 1) x (-1, 0, 0)
  line L0 (17.4, 13) -> (-17.4, 13)
  line L1 (-17.4, 13) -> (-17.4, 15)
  line L2 (-17.4, 15) -> (-31, 15)
  line L3 (-31, 15) -> (-31, 9)
  line L4 (-31, 9) -> (-29, 9)
  line L5 (-29, 9) -> (-29, 3)
  line L6 (-29, 3) -> (-31, 3)
  line L7 (-31, 3) -> (-31, -3)
  line L8 (-31, -3) -> (-29, -3)
  line L9 (-29, -3) -> (-29, -9)
  line L10 (-29, -9) -> (-31, -9)
  line L11 (-31, -9) -> (-31, -15)
  line L12 (-31, -15) -> (-17.4, -15)
  line L13 (-17.4, -15) -> (-17.4, -13)
  line L14 (-17.4, -13) -> (-5.8, -13)
  line L15 (-5.8, -13) -> (-5.8, -15)
  line L16 (-5.8, -15) -> (5.8, -15)
  line L17 (5.8, -15) -> (5.8, -13)
  line L18 (5.8, -13) -> (17.4, -13)
  line L19 (17.4, -13) -> (17.4, -15)
  line L20 (17.4, -15) -> (31, -15)
  line L21 (31, -15) -> (31, -9)
  line L22 (31, -9) -> (29, -9)
  line L23 (29, -9) -> (29, -3)
  line L24 (29, -3) -> (31, -3)
  line L25 (31, -3) -> (31, 3)
  line L26 (31, 3) -> (29, 3)
  line L27 (29, 3) -> (29, 9)
  line L28 (29, 9) -> (31, 9)
  line L29 (31, 9) -> (31, 15)
  line L30 (31, 15) -> (17.4, 15)
  line L31 (17.4, 15) -> (17.4, 13)
  line L32 (11, 0) -> (-27, 0)
  line L33 (-27, 0) -> (-27, 5)
  line L34 (-27, 5) -> (11, 5)
  line L35 (11, 5) -> (11, 0)
  dimension "d26" = 2
  dimension "d27" = 40
  dimension "d28" = 5
  dimension "d29" = 8
  constraint horizontal L32
  constraint vertical L33
  constraint horizontal L34
  constraint vertical L35
  measures "d26" distance of L5 L33
  measures "d27" distance of L5 L35
  measures "d28" distance of L32.start L34.end
  measures "d29" distance of L0 L34
extrude "押し出し5" cut sketch "スケッチ5" against normal up to surface (2 mm away) contours L32 L33 L34 L35
extrude "押し出し6" cut 1 faces at (-5.8, -13, 1.3333) along direction (0, 1, 0) blind 2
equation "d1 = 58 mm + t * 2"
equation "d3 = t"
equation "t = 2 mm" comment "板厚"
equation "w = 11.6 mm" comment "かみ合い幅"
equation "d9 = w3"
equation "d10 = w3 / 2"
equation "w2 = 18 mm"
equation "w3 = 6 mm"
equation "d16 = w"
equation "d21 = t"
equation "d22 = w / 2"
equation "d23 = t"
equation "d24 = -t"

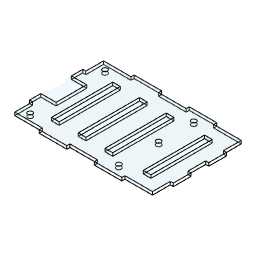
design "teimen"
Autodesk Fusion 360 part; units mm, degrees
sketch "スケッチ1" plane through (0, 0, 0) normal (0, 0, 1) x (1, 0, 0)
  line L0 (45, 29) -> (-45, 29)
  line L1 (-45, 29) -> (-45, -29)
  line L2 (-45, -29) -> (45, -29)
  line L3 (45, -29) -> (45, 29)
  line L4 (45, 29) -> (-45, -29) construction
  line L5 (-45, 29) -> (45, -29) construction
  dimension "d1" = 90
  dimension "d2" = 58
  constraint horizontal L0
  constraint perpendicular L0 L1
  constraint parallel L0 L2
  constraint parallel L1 L3
  constraint coincident L4 origin
  constraint coincident L5 origin
  measures "d1" distance of L0.start L0.end
  measures "d2" distance of L0.end L1.end
extrude "押し出し1" add sketch "スケッチ1" along normal blind 2
sketch "スケッチ2" plane through (0, 0, 0) normal (0, 0, 1) x (1, 0, 0)
  line L0 (45, 17.4) -> (47, 17.4)
  line L1 (47, 17.4) -> (47, 5.8)
  line L2 (47, 5.8) -> (45, 5.8)
  line L3 (45, 5.8) -> (45, 17.4)
  line L4 (45, -29) -> (45, 29)
  line L5 (0, 0) -> (48, 0)
  line L6 (45, -5.8) -> (45, -17.4)
  line L7 (47, -5.8) -> (45, -5.8)
  line L8 (47, -17.4) -> (47, -5.8)
  line L9 (45, -17.4) -> (47, -17.4)
  line L10 (0, 0) -> (0, -25)
  line L11 (-45, 17.4) -> (-47, 17.4)
  line L12 (-45, 5.8) -> (-45, 17.4)
  line L13 (-47, -5.8) -> (-45, -5.8)
  line L14 (-45, -5.8) -> (-45, -17.4)
  line L15 (-45, -17.4) -> (-47, -17.4)
  line L16 (-47, -17.4) -> (-47, -5.8)
  line L17 (-47, 5.8) -> (-45, 5.8)
  line L18 (-47, 17.4) -> (-47, 5.8)
  dimension "d6" = 2
  dimension "d9" = 11.6
  dimension "d10" = 5.8
  constraint horizontal L0
  constraint vertical L1
  constraint horizontal L2
  constraint vertical L3
  constraint collinear L3 L4
  constraint coincident L5.start L10.start
  constraint perpendicular L4 L5
  constraint symmetric L0.start L5 L6.end
  constraint symmetric L0.end L5 L8.start
  constraint symmetric L1.end L5 L7.start
  constraint symmetric L2.end L5 L6.start
  constraint perpendicular L5 L10
  constraint symmetric L0.start L10 L11.start
  constraint symmetric L0.end L10 L11.end
  constraint symmetric L1.end L10 L17.start
  constraint symmetric L2.end L10 L12.start
  constraint symmetric L8.start L10 L15.end
  constraint symmetric L6.end L10 L14.end
  constraint symmetric L6.start L10 L13.end
  constraint symmetric L7.start L10 L13.start
  measures "d6" distance of L0.start L0.end
  measures "d9" distance of L0.end L1.end
  measures "d10" distance of L5.start L2
extrude "押し出し2" add sketch "スケッチ2" along normal up to surface (2 mm away)
sketch "スケッチ3" plane through (0, 0, 2) normal (0, 0, 1) x (-1, 0, 0)
  line L0 (-45, 29) -> (-45, 17.4)
  line L1 (-45, 17.4) -> (-47, 17.4)
  line L2 (-47, 17.4) -> (-47, 5.8)
  line L3 (-47, 5.8) -> (-45, 5.8)
  line L4 (-45, 5.8) -> (-45, -5.8)
  line L5 (-45, -5.8) -> (-47, -5.8)
  line L6 (-47, -5.8) -> (-47, -17.4)
  line L7 (-47, -17.4) -> (-45, -17.4)
  line L8 (-45, -17.4) -> (-45, -29)
  line L9 (-45, -29) -> (45, -29)
  line L10 (45, -29) -> (45, -17.4)
  line L11 (45, -17.4) -> (47, -17.4)
  line L12 (47, -17.4) -> (47, -5.8)
  line L13 (47, -5.8) -> (45, -5.8)
  line L14 (45, -5.8) -> (45, 5.8)
  line L15 (45, 5.8) -> (47, 5.8)
  line L16 (47, 5.8) -> (47, 17.4)
  line L17 (47, 17.4) -> (45, 17.4)
  line L18 (45, 17.4) -> (45, 29)
  line L19 (45, 29) -> (-45, 29)
  line L20 (27, -29) -> (9, -29)
  line L21 (9, -29) -> (9, -31)
  line L22 (9, -31) -> (27, -31)
  line L23 (27, -31) -> (27, -29)
  line L24 (0, 0) -> (0, -29)
  line L25 (-27, -31) -> (-27, -29)
  line L26 (-9, -31) -> (-27, -31)
  line L27 (-9, -29) -> (-9, -31)
  line L28 (-27, -29) -> (-9, -29)
  line L29 (0, 0) -> (45, 0)
  line L30 (9, 31) -> (27, 31)
  line L31 (-27, 29) -> (-9, 29)
  line L32 (9, 29) -> (9, 31)
  line L33 (-27, 31) -> (-27, 29)
  line L34 (27, 29) -> (9, 29)
  line L35 (-9, 29) -> (-9, 31)
  line L36 (-9, 31) -> (-27, 31)
  line L37 (27, 31) -> (27, 29)
  point P0 (0, 29)
  dimension "d16" = 18
  dimension "d17" = 9
  dimension "d18" = 2
  constraint horizontal L20
  constraint vertical L21
  constraint horizontal L22
  constraint vertical L23
  constraint coincident L9 L20.start
  constraint coincident L24.start L29.start
  constraint midpoint L9 L24.end
  constraint symmetric L20.start L24 L25.end
  constraint symmetric L20.end L24 L27.start
  constraint symmetric L21.end L24 L26.start
  constraint symmetric L22.end L24 L25.start
  constraint midpoint L14 L29.end
  constraint symmetric L20.start L29 L34.start
  constraint symmetric L20.end L29 L32.start
  constraint symmetric L21.end L29 L30.start
  constraint symmetric L22.end L29 L30.end
  constraint symmetric L24.end L29 P0
  constraint symmetric L26.start L29 L35.end
  constraint symmetric L27.start L29 L31.end
  constraint symmetric L25.start L29 L33.start
  constraint symmetric L25.end L29 L31.start
  measures "d16" distance of L21.end L22.end
  measures "d17" distance of L24.start L21
  measures "d18" distance of L20.start L22.end
extrude "押し出し3" add sketch "スケッチ3" against normal up to surface (2 mm away) contours L19 L31 L33 L35 L36 | L19 L30 L32 L34 L37 | L9 L25 L26 L27 L28 | L9 L20 L21 L22 L23
sketch "スケッチ4" plane through (0, 0, 2) normal (0, 0, 1) x (-1, 0, 0)
  line L0 (-45, 29) -> (-45, 17.4)
  line L1 (-45, 17.4) -> (-47, 17.4)
  line L2 (-47, 17.4) -> (-47, 5.8)
  line L3 (-47, 5.8) -> (-45, 5.8)
  line L4 (-45, 5.8) -> (-45, -5.8)
  line L5 (-45, -5.8) -> (-47, -5.8)
  line L6 (-47, -5.8) -> (-47, -17.4)
  line L7 (-47, -17.4) -> (-45, -17.4)
  line L8 (-45, -17.4) -> (-45, -29)
  line L9 (-45, -29) -> (-27, -29)
  line L10 (-27, -29) -> (-27, -31)
  line L11 (-27, -31) -> (-9, -31)
  line L12 (-9, -31) -> (-9, -29)
  line L13 (-9, -29) -> (9, -29)
  line L14 (9, -29) -> (9, -31)
  line L15 (9, -31) -> (27, -31)
  line L16 (27, -31) -> (27, -29)
  line L17 (27, -29) -> (45, -29)
  line L18 (45, -29) -> (45, -17.4)
  line L19 (45, -17.4) -> (47, -17.4)
  line L20 (47, -17.4) -> (47, -5.8)
  line L21 (47, -5.8) -> (45, -5.8)
  line L22 (45, -5.8) -> (45, 5.8)
  line L23 (45, 5.8) -> (47, 5.8)
  line L24 (47, 5.8) -> (47, 17.4)
  line L25 (47, 17.4) -> (45, 17.4)
  line L26 (45, 17.4) -> (45, 29)
  line L27 (45, 29) -> (27, 29)
  line L28 (27, 29) -> (27, 31)
  line L29 (27, 31) -> (9, 31)
  line L30 (9, 31) -> (9, 29)
  line L31 (9, 29) -> (-9, 29)
  line L32 (-9, 29) -> (-9, 31)
  line L33 (-9, 31) -> (-27, 31)
  line L34 (-27, 31) -> (-27, 29)
  line L35 (-27, 29) -> (-45, 29)
sketch "スケッチ5" plane through (0, 0, 2) normal (0, 0, 1) x (1, 0, 0)
  line L0 (-37, -10) -> (-47, -10)
  line L1 (-47, -10) -> (-47, 10)
  line L2 (-47, 10) -> (-37, 10)
  line L3 (-37, 10) -> (-37, -10)
  line L4 (47, -17.4) -> (47, -5.8)
  line L5 (-47, 17.4) -> (-47, 5.8)
  dimension "d21" = 20
  dimension "d22" = 10
  dimension "d23" = 10
  constraint horizontal L0
  constraint vertical L1
  constraint horizontal L2
  constraint vertical L3
  constraint collinear L1 L5
  measures "d21" distance of L0.start L2.end
  measures "d22" distance of origin L0
  measures "d23" distance of L0.start L0.end
extrude "押し出し4" cut sketch "スケッチ5" against normal blind 2
sketch "スケッチ6" plane through (0, 0, 2) normal (0, 0, 1) x (-1, 0, 0)
  circle A0 centre (-18.5, 24.5) radius 1.6
  circle A1 centre (39.5, 24.5) radius 1.6
  circle A2 centre (-18.5, -24.5) radius 1.6
  circle A3 centre (39.5, -24.5) radius 1.6
  line L0 (45, 17.4) -> (45, 29)
  circle A4 centre (-18.5, -1.5) radius 1.6
  dimension "d26" = 3.2
  dimension "d29" = 58
  dimension "d30" = -49
  dimension "d31" = 24.5
  dimension "d32" = 5.5
  dimension "d37" = 15
  dimension "d38" = 23
  measures "d26" diameter of A0
  measures "d31" vertical distance of origin A0.centre
  measures "d32" distance of A1.centre L0
extrude "押し出し5" cut sketch "スケッチ6" against normal up to surface (2 mm away)
sketch "スケッチ7" plane through (0, 0, 2) normal (0, 0, 1) x (-1, 0, 0)
sketch "スケッチ8" plane through (0, 0, 2) normal (0, 0, 1) x (1, 0, 0)
  line L0 (10, -20) -> (5, -20)
  line L1 (5, -20) -> (5, 20)
  line L2 (5, 20) -> (10, 20)
  line L3 (10, 20) -> (10, -20)
  line L4 (-12.5, -20) -> (-12.5, 20)
  line L5 (-7.5, 20) -> (-7.5, -20)
  line L6 (-7.5, -20) -> (-12.5, -20)
  line L7 (-12.5, 20) -> (-7.5, 20)
  line L8 (-30, -20) -> (-30, 20)
  line L9 (-25, 20) -> (-25, -20)
  line L10 (-25, -20) -> (-30, -20)
  line L11 (-30, 20) -> (-25, 20)
  line L12 (35, 20) -> (35, -20)
  line L13 (30, 20) -> (35, 20)
  line L14 (35, -20) -> (30, -20)
  line L15 (30, -20) -> (30, 20)
  dimension "d41" = -35
  dimension "d42" = 0
  dimension "d45" = 25
  dimension "d46" = 0
  constraint horizontal L0
  constraint vertical L1
  constraint horizontal L2
  constraint vertical L3
extrude "押し出し6" cut sketch "スケッチ8" against normal up to surface (2 mm away)
equation "d3 = t"
equation "t = 2 mm" comment "板厚"
equation "d6 = t"
equation "w = 11.6 mm" comment "かみ合い幅"
equation "d9 = w"
equation "d10 = w / 2"
equation "w2 = 18 mm"
equation "w3 = 6 mm"
equation "d16 = w2"
equation "d17 = w2 / 2"
equation "d18 = t"
equation "d24 = -t"
equation "d31 = ( 49 / 2 ) * 1 mm"

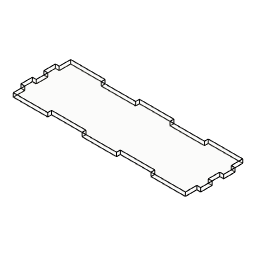
design "haimen"
Autodesk Fusion 360 part; units mm, degrees
sketch "スケッチ1" plane through (0, 0, 0) normal (0, 0, 1) x (1, 0, 0)
  line L0 (45, 15) -> (-45, 15)
  line L1 (-45, 15) -> (-45, -15)
  line L2 (-45, -15) -> (45, -15)
  line L3 (45, -15) -> (45, 15)
  line L4 (45, 15) -> (-45, -15) construction
  line L5 (-45, 15) -> (45, -15) construction
  dimension "d1" = 90
  dimension "d2" = 30
  constraint horizontal L0
  constraint perpendicular L0 L1
  constraint parallel L0 L2
  constraint parallel L1 L3
  constraint coincident L4 origin
  constraint coincident L5 origin
  measures "d1" distance of L0.start L0.end
  measures "d2" distance of L0.end L1.end
extrude "押し出し1" add sketch "スケッチ1" along normal blind 2
sketch "スケッチ2" plane through (0, 0, 0) normal (0, 0, 1) x (1, 0, 0)
  line L0 (45, 9) -> (47, 9)
  line L1 (47, 9) -> (47, 3)
  line L2 (47, 3) -> (45, 3)
  line L3 (45, 3) -> (45, 9)
  line L4 (45, -15) -> (45, 15)
  line L5 (0, 0) -> (48, 0)
  line L6 (45, -3) -> (45, -9)
  line L7 (47, -3) -> (45, -3)
  line L8 (47, -9) -> (47, -3)
  line L9 (45, -9) -> (47, -9)
  line L10 (0, 0) -> (0, -25)
  line L11 (-45, 9) -> (-47, 9)
  line L12 (-45, 3) -> (-45, 9)
  line L13 (-47, -3) -> (-45, -3)
  line L14 (-45, -3) -> (-45, -9)
  line L15 (-45, -9) -> (-47, -9)
  line L16 (-47, -9) -> (-47, -3)
  line L17 (-47, 3) -> (-45, 3)
  line L18 (-47, 9) -> (-47, 3)
  dimension "d6" = 2
  dimension "d9" = 6
  dimension "d10" = 3
  constraint horizontal L0
  constraint vertical L1
  constraint horizontal L2
  constraint vertical L3
  constraint collinear L3 L4
  constraint coincident L5.start L10.start
  constraint perpendicular L4 L5
  constraint symmetric L0.start L5 L6.end
  constraint symmetric L0.end L5 L8.start
  constraint symmetric L1.end L5 L7.start
  constraint symmetric L2.end L5 L6.start
  constraint perpendicular L5 L10
  constraint symmetric L0.start L10 L11.start
  constraint symmetric L0.end L10 L11.end
  constraint symmetric L1.end L10 L17.start
  constraint symmetric L2.end L10 L12.start
  constraint symmetric L8.start L10 L15.end
  constraint symmetric L6.end L10 L14.end
  constraint symmetric L6.start L10 L13.end
  constraint symmetric L7.start L10 L13.start
  measures "d6" distance of L0.start L0.end
  measures "d9" distance of L0.end L1.end
  measures "d10" distance of L5.start L2
extrude "押し出し2" add sketch "スケッチ2" along normal up to surface (2 mm away)
sketch "スケッチ3" plane through (0, 0, 2) normal (0, 0, 1) x (-1, 0, 0)
  line L0 (-45, 9) -> (-47, 9)
  line L1 (-47, 9) -> (-47, 3)
  line L2 (-47, 3) -> (-45, 3)
  line L3 (-45, 15) -> (-45, 9)
  line L4 (-45, -3) -> (-47, -3)
  line L5 (-47, -3) -> (-47, -9)
  line L6 (-47, -9) -> (-45, -9)
  line L7 (-45, -15) -> (45, -15)
  line L8 (45, -9) -> (47, -9)
  line L9 (47, -9) -> (47, -3)
  line L10 (47, -3) -> (45, -3)
  line L11 (45, -15) -> (45, -9)
  line L12 (45, 3) -> (47, 3)
  line L13 (47, 3) -> (47, 9)
  line L14 (47, 9) -> (45, 9)
  line L15 (27, -15) -> (9, -15)
  line L16 (9, -15) -> (9, -13)
  line L17 (9, -13) -> (27, -13)
  line L18 (27, -13) -> (27, -15)
  line L19 (-45, -9) -> (-45, -15)
  line L20 (45, 9) -> (45, 15)
  line L21 (0, 0) -> (0, -10)
  line L22 (0, 0) -> (9, 0)
  line L23 (-27, -15) -> (-9, -15)
  line L24 (-9, -15) -> (-9, -13)
  line L25 (-27, -13) -> (-27, -15)
  line L26 (-9, -13) -> (-27, -13)
  line L27 (-9, 15) -> (-9, 13)
  line L28 (-27, 13) -> (-27, 15)
  line L29 (27, 15) -> (9, 15)
  line L30 (9, 13) -> (27, 13)
  line L31 (-27, 15) -> (-9, 15)
  line L32 (-9, 13) -> (-27, 13)
  line L33 (9, 15) -> (9, 13)
  line L34 (27, 13) -> (27, 15)
  line L35 (-45, 3) -> (-45, -3)
  line L36 (45, -3) -> (45, 3)
  dimension "d16" = 18
  dimension "d21" = 2
  dimension "d22" = 9
  constraint horizontal L15
  constraint vertical L16
  constraint horizontal L17
  constraint vertical L18
  constraint coincident L7 L15.start
  constraint coincident L21.start L22.start
  constraint parallel L16 L21
  constraint perpendicular L21 L22
  constraint symmetric L15.start L21 L23.start
  constraint symmetric L15.end L21 L23.end
  constraint symmetric L16.end L21 L24.end
  constraint symmetric L17.end L21 L25.start
  constraint symmetric L15.start L22 L29.start
  constraint symmetric L15.end L22 L29.end
  constraint symmetric L16.end L22 L30.start
  constraint symmetric L17.end L22 L30.end
  constraint symmetric L22 L23.start L28.end
  constraint symmetric L22 L23.end L27.start
  constraint symmetric L22 L25.start L28.start
  constraint symmetric L22 L24.end L27.end
  measures "d16" distance of L16.end L17.end
  measures "d21" distance of L7 L17
  measures "d22" distance of L21.start L16
extrude "押し出し3" cut sketch "スケッチ3" against normal up to surface (2 mm away)
equation "d3 = t"
equation "t = 2 mm" comment "板厚"
equation "d6 = t"
equation "w = 11.6 mm" comment "かみ合い幅"
equation "d9 = w3"
equation "d10 = w3 / 2"
equation "w2 = 18 mm"
equation "w3 = 6 mm"
equation "d16 = w2"
equation "d21 = t"
equation "d22 = w2 / 2"

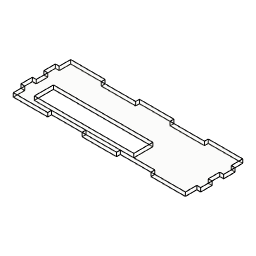
design "zenmen"
Autodesk Fusion 360 part; units mm, degrees
sketch "スケッチ1" plane through (0, 0, 0) normal (0, 0, 1) x (1, 0, 0)
  line L0 (45, 15) -> (-45, 15)
  line L1 (-45, 15) -> (-45, -15)
  line L2 (-45, -15) -> (45, -15)
  line L3 (45, -15) -> (45, 15)
  line L4 (45, 15) -> (-45, -15) construction
  line L5 (-45, 15) -> (45, -15) construction
  dimension "d1" = 90
  dimension "d2" = 30
  constraint horizontal L0
  constraint perpendicular L0 L1
  constraint parallel L0 L2
  constraint parallel L1 L3
  constraint coincident L4 origin
  constraint coincident L5 origin
  measures "d1" distance of L0.start L0.end
  measures "d2" distance of L0.end L1.end
extrude "押し出し1" add sketch "スケッチ1" along normal blind 2
sketch "スケッチ2" plane through (0, 0, 0) normal (0, 0, 1) x (1, 0, 0)
  line L0 (45, 9) -> (47, 9)
  line L1 (47, 9) -> (47, 3)
  line L2 (47, 3) -> (45, 3)
  line L3 (45, 3) -> (45, 9)
  line L4 (45, -15) -> (45, 15)
  line L5 (0, 0) -> (48, 0)
  line L6 (45, -3) -> (45, -9)
  line L7 (47, -3) -> (45, -3)
  line L8 (47, -9) -> (47, -3)
  line L9 (45, -9) -> (47, -9)
  line L10 (0, 0) -> (0, -25)
  line L11 (-45, 9) -> (-47, 9)
  line L12 (-45, 3) -> (-45, 9)
  line L13 (-47, -3) -> (-45, -3)
  line L14 (-45, -3) -> (-45, -9)
  line L15 (-45, -9) -> (-47, -9)
  line L16 (-47, -9) -> (-47, -3)
  line L17 (-47, 3) -> (-45, 3)
  line L18 (-47, 9) -> (-47, 3)
  dimension "d6" = 2
  dimension "d9" = 6
  dimension "d10" = 3
  constraint horizontal L0
  constraint vertical L1
  constraint horizontal L2
  constraint vertical L3
  constraint collinear L3 L4
  constraint coincident L5.start L10.start
  constraint perpendicular L4 L5
  constraint symmetric L0.start L5 L6.end
  constraint symmetric L0.end L5 L8.start
  constraint symmetric L1.end L5 L7.start
  constraint symmetric L2.end L5 L6.start
  constraint perpendicular L5 L10
  constraint symmetric L0.start L10 L11.start
  constraint symmetric L0.end L10 L11.end
  constraint symmetric L1.end L10 L17.start
  constraint symmetric L2.end L10 L12.start
  constraint symmetric L8.start L10 L15.end
  constraint symmetric L6.end L10 L14.end
  constraint symmetric L6.start L10 L13.end
  constraint symmetric L7.start L10 L13.start
  measures "d6" distance of L0.start L0.end
  measures "d9" distance of L0.end L1.end
  measures "d10" distance of L5.start L2
extrude "押し出し2" add sketch "スケッチ2" along normal up to surface (2 mm away)
sketch "スケッチ3" plane through (0, 0, 2) normal (0, 0, 1) x (-1, 0, 0)
  line L0 (-45, 9) -> (-47, 9)
  line L1 (-47, 9) -> (-47, 3)
  line L2 (-47, 3) -> (-45, 3)
  line L3 (-45, 15) -> (-45, 9)
  line L4 (-45, -3) -> (-47, -3)
  line L5 (-47, -3) -> (-47, -9)
  line L6 (-47, -9) -> (-45, -9)
  line L7 (-45, -15) -> (45, -15)
  line L8 (45, -9) -> (47, -9)
  line L9 (47, -9) -> (47, -3)
  line L10 (47, -3) -> (45, -3)
  line L11 (45, -15) -> (45, -9)
  line L12 (45, 3) -> (47, 3)
  line L13 (47, 3) -> (47, 9)
  line L14 (47, 9) -> (45, 9)
  line L15 (27, -15) -> (9, -15)
  line L16 (9, -15) -> (9, -13)
  line L17 (9, -13) -> (27, -13)
  line L18 (27, -13) -> (27, -15)
  line L19 (-45, -9) -> (-45, -15)
  line L20 (45, 9) -> (45, 15)
  line L21 (0, 0) -> (0, -10)
  line L22 (0, 0) -> (9, 0)
  line L23 (-27, -15) -> (-9, -15)
  line L24 (-9, -15) -> (-9, -13)
  line L25 (-27, -13) -> (-27, -15)
  line L26 (-9, -13) -> (-27, -13)
  line L27 (-9, 15) -> (-9, 13)
  line L28 (-27, 13) -> (-27, 15)
  line L29 (27, 15) -> (9, 15)
  line L30 (9, 13) -> (27, 13)
  line L31 (-27, 15) -> (-9, 15)
  line L32 (-9, 13) -> (-27, 13)
  line L33 (9, 15) -> (9, 13)
  line L34 (27, 13) -> (27, 15)
  line L35 (-45, 3) -> (-45, -3)
  line L36 (45, -3) -> (45, 3)
  dimension "d16" = 18
  dimension "d21" = 2
  dimension "d22" = 9
  constraint horizontal L15
  constraint vertical L16
  constraint horizontal L17
  constraint vertical L18
  constraint coincident L7 L15.start
  constraint coincident L21.start L22.start
  constraint parallel L16 L21
  constraint perpendicular L21 L22
  constraint symmetric L15.start L21 L23.start
  constraint symmetric L15.end L21 L23.end
  constraint symmetric L16.end L21 L24.end
  constraint symmetric L17.end L21 L25.start
  constraint symmetric L15.start L22 L29.start
  constraint symmetric L15.end L22 L29.end
  constraint symmetric L16.end L22 L30.start
  constraint symmetric L17.end L22 L30.end
  constraint symmetric L22 L23.start L28.end
  constraint symmetric L22 L23.end L27.start
  constraint symmetric L22 L25.start L28.start
  constraint symmetric L22 L24.end L27.end
  measures "d16" distance of L16.end L17.end
  measures "d21" distance of L7 L17
  measures "d22" distance of L21.start L16
extrude "押し出し3" cut sketch "スケッチ3" against normal up to surface (2 mm away)